20mm tooling (Autodesk Fusion 360 design; units mm, degrees)
Autodesk Fusion 360 part; units mm, degrees
note: some values were not read from the file. Chosen so that the rebuilt part matches the saved one: which pieces of a blend or face edit are solid. Set by a fixed rule: which sketch regions a step uses.
sketch "Sketch1" plane through (0, 0, 0) normal (0, 1, 0) x (1, 0, 0)
  line L0 (0, 0) -> (144, 0)
  line L1 (144, -40) -> (0, -40)
  line L2 (0, -40) -> (0, 0)
  line L3 (0, -20) -> (144, -20)
  line L4 (0, 0) -> (10, 0)
  line L5 (144, 0) -> (140, 0)
  line L6 (10, 0) -> (36, 0)
  line L7 (36, -40) -> (62, -40)
  line L8 (62, 0) -> (88, 0)
  line L9 (88, -40) -> (114, -40)
  line L10 (114, 0) -> (140, 0)
  circle A0 centre (20, -20) radius 10
  circle A1 centre (46, -20) radius 10
  circle A2 centre (72, -20) radius 10
  circle A3 centre (124, -20) radius 10
  line L11 (134, -20) -> (144, -20)
  line L12 (144, -40) -> (144, 0)
  circle A4 centre (98, -20) radius 10
  line L13 (0, 0) -> (144, 0)
  line L14 (144, 0) -> (144, -5)
  line L15 (144, -5) -> (0, -5)
  line L16 (0, -5) -> (0, 0)
  line L17 (0, -40) -> (5, -40)
  line L18 (5, -40) -> (5, 0)
  line L19 (5, 0) -> (0, 0)
  line L20 (0, 0) -> (0, -40)
  line L21 (144, -40) -> (139, -40)
  line L22 (139, -40) -> (139, 0)
  line L23 (139, 0) -> (144, 0)
  line L24 (144, 0) -> (144, -40)
  dimension "d8" = 20
  dimension "d9" = 20
  dimension "d10" = 20
  dimension "d12" = 20
  dimension "d15" = 20
  dimension "d16" = 5
  dimension "d17" = 5
  constraint horizontal L0
  constraint horizontal L1
  constraint vertical L2
  constraint coincident L0.start L2.end
  constraint midpoint L2 L3.start
  constraint coincident L0 L4.end
  constraint perpendicular L2 L4
  constraint coincident L0 L5.end
  constraint coincident L1 L7.start
  constraint coincident L0 L8.start
  constraint coincident L1 L9.start
  constraint coincident L0 L10.start
  constraint coincident A3 L11.start
  constraint coincident L3 L11.start
  constraint coincident L1 L12.start
  constraint vertical L12
  constraint horizontal L13
  constraint vertical L14
  constraint horizontal L15
  constraint vertical L16
  constraint horizontal L17
  constraint vertical L18
  constraint horizontal L19
  constraint vertical L20
  constraint midpoint L4 L18.end
  constraint horizontal L21
  constraint vertical L22
  constraint horizontal L23
  constraint vertical L24
  measures "d8" diameter of A0
  measures "d9" diameter of A1
  measures "d10" diameter of A2
  measures "d12" diameter of A3
  measures "d15" diameter of A4
  measures "d16" distance of L0.start L15.end
  measures "d17" distance of L1.start L21.end
extrude "Extrude1" add sketch "Sketch1" along normal blind 5 contours L0 L2 L4 L13 L15 L16 L18 L19 L20 | L0 L4 L6 L8 L10 L13 L15 L18 L22 | L2 L3 L15 L18 L20 | L3 A0 A1 A2 A3 L11 A4 L15 L18 L22 | L1 L2 L3 L17 L18 L20 | L0 L5 L10 L12 L13 L14 L15 L22 L23 L24 | L3 L11 L12 L15 L22 L24 | L1 L3 L7 L9 A0 A1 A2 A3 L11 A4 L18 L22 | L1 L3 L11 L12 L21 L22 L24
fillet "Fillet1" radius 2 10 edges at (10.6767, 5, 16.3838) (36.6767, 5, 16.3838) (62.6767, 5, 16.3838) (88.6767, 5, 16.3838) (114.6767, 5, 16.3838) (10.6767, 0, 16.3838) (36.6767, 0, 16.3838) (62.6767, 0, 16.3838) (88.6767, 0, 16.3838) (114.6767, 0, 16.3838)
fillet "Fillet2" radius 2 2 edges at (72, 5, 40) (72, 0, 40)
sketch "Sketch2" plane through (0, 0, 0) normal (0, -1, 0) x (1, 0, 0)
  circle A0 centre (124, 20) radius 12
  circle A1 centre (72, 20) radius 12
  circle A2 centre (20, 20) radius 12
  line L0 (144, 38) -> (0, 38)
  line L1 (0, 38) -> (0, 0)
  line L2 (0, 0) -> (144, 0)
  line L3 (144, 0) -> (144, 38)
  circle A3 centre (46, 20) radius 12
  circle A4 centre (98, 20) radius 12
  line L4 (0, 0) -> (144, 0)
  line L5 (144, 0) -> (144, 5)
  line L6 (144, 5) -> (0, 5)
  line L7 (0, 5) -> (0, 0)
  line L8 (0, 0) -> (5, 0)
  line L9 (5, 0) -> (5, 38)
  line L10 (5, 38) -> (0, 38)
  line L11 (0, 38) -> (0, 0)
  line L12 (144, 0) -> (139, 0)
  line L13 (139, 0) -> (139, 38)
  line L14 (139, 38) -> (144, 38)
  line L15 (144, 38) -> (144, 0)
  dimension "d22" = 5
  dimension "d23" = 5
  dimension "d24" = 5
  constraint horizontal L4
  constraint vertical L5
  constraint horizontal L6
  constraint vertical L7
  constraint coincident L1.end L2.start
  constraint horizontal L8
  constraint vertical L9
  constraint horizontal L10
  constraint vertical L11
  constraint horizontal L12
  constraint vertical L13
  constraint horizontal L14
  constraint vertical L15
  measures "d22" distance of L1.end L6.end
  measures "d23" distance of L1.end L8.end
  measures "d24" distance of L2.end L12.end
extrude "Extrude2" add sketch "Sketch2" along normal blind 5 contours L0 L3 L6 L13 L14 L15 | L2 L3 L4 L5 L6 L12 L13 L15 | L0 L1 L6 L9 L10 L11 | L2 L4 L6 L9 L13 | L1 L2 L4 L6 L7 L8 L9 L11
fillet "Fillet3" radius 100 2 edges at (2.5, -5, 38) (141.5, -5, 38)
sketch "Sketch3" plane through (0, -5, 0) normal (0, -1, 0) x (1, 0, 0)
  line L0 (144, 6.775) -> (139, 6.775)
  line L1 (139, 6.775) -> (139, 5)
  line L2 (139, 5) -> (5, 5)
  line L3 (5, 5) -> (5, 6.775)
  line L4 (5, 6.775) -> (0, 6.775)
  line L5 (0, 6.775) -> (0, 0)
  line L6 (0, 0) -> (144, 0)
  line L7 (144, 0) -> (144, 6.775)
  line L8 (72, 0) -> (72, 5)
  line L9 (72, 5) -> (82, 5)
  line L10 (82, 5) -> (82, 0)
  line L11 (82, 0) -> (72, 0)
  line L12 (72, 0) -> (72, 5)
  line L13 (72, 0) -> (62, 0)
  line L14 (62, 0) -> (62, 5)
  line L15 (62, 5) -> (72, 5)
  line L16 (72, 5) -> (72, 0)
  line L17 (5, 5) -> (25, 5)
  line L18 (25, 5) -> (25, 0)
  line L19 (25, 0) -> (5, 0)
  line L20 (5, 0) -> (5, 5)
  line L21 (139, 5) -> (119, 5)
  line L22 (119, 5) -> (119, 0)
  line L23 (119, 0) -> (139, 0)
  line L24 (139, 0) -> (139, 5)
  dimension "d28" = 10
  dimension "d29" = 10
  dimension "d30" = 20
  dimension "d31" = 20
  constraint midpoint L6 L8.start
  constraint midpoint L2 L8.end
  constraint horizontal L9
  constraint vertical L10
  constraint horizontal L11
  constraint vertical L12
  constraint horizontal L13
  constraint vertical L14
  constraint horizontal L15
  constraint vertical L16
  constraint horizontal L17
  constraint vertical L18
  constraint horizontal L19
  constraint vertical L20
  constraint coincident L2.end L3.start
  constraint horizontal L21
  constraint vertical L22
  constraint horizontal L23
  constraint vertical L24
  constraint coincident L1.end L2.start
  measures "d28" distance of L8.end L9.end
  measures "d29" distance of L8.start L13.end
  measures "d30" distance of L2.end L17.end
  measures "d31" distance of L1.end L21.end
extrude "Extrude3" add sketch "Sketch3" along normal blind 10 contours L2 L6 L21 L22 L23 L24 | L2 L6 L8 L9 L10 L11 L12 L16 | L2 L6 L8 L12 L13 L14 L15 L16 | L2 L6 L17 L18 L19 L20
fillet "Fillet4" radius 10 6 edges at (5, -15, 2.5) (25, -15, 2.5) (62, -15, 2.5) (82, -15, 2.5) (119, -15, 2.5) (139, -15, 2.5)
sketch "Sketch4" plane through (0, 0, 5) normal (0, 0, 1) x (1, 0, 0)
  arc A0 (119, -5) -> (139, -5) centre (129, -5) ccw
  line L0 (139, -5) -> (139, 0)
  line L1 (139, 0) -> (5, 0)
  line L2 (5, 0) -> (5, -5)
  arc A1 (5, -5) -> (25, -5) centre (15, -5) ccw
  line L3 (25, -5) -> (62, -5)
  arc A2 (62, -5) -> (82, -5) centre (72, -5) ccw
  line L4 (82, -5) -> (119, -5)
  line L5 (15, -15) -> (15, 0)
  line L6 (72, -15) -> (72, 0)
  line L7 (129, -15) -> (129, 0)
  line L8 (5, -5) -> (139, -5)
  circle A3 centre (15, -5) radius 1.5
  circle A4 centre (10, -5) radius 1.5
  circle A5 centre (20, -5) radius 1.5
  circle A6 centre (72, -5) radius 1.5
  line L9 (62, -5) -> (82, -5)
  line L10 (62, -5) -> (67, -5)
  line L11 (82, -5) -> (77, -5)
  circle A7 centre (67, -5) radius 1.5
  circle A8 centre (77, -5) radius 1.5
  line L12 (119, -5) -> (139, -5)
  circle A9 centre (129, -5) radius 1.5
  line L13 (119, -5) -> (129, -5)
  circle A10 centre (124, -5) radius 1.5
  line L14 (139, -5) -> (129, -5)
  circle A11 centre (134, -5) radius 1.5
  line L15 (72, -5) -> (72, -15)
  circle A12 centre (72, -10) radius 1.5
  line L16 (15, -15) -> (15, -5)
  circle A13 centre (15, -10) radius 1.5
  line L17 (129, -15) -> (129, -5)
  circle A14 centre (129, -10) radius 1.5
  circle A15 centre (15, 0) radius 1.5
  circle A16 centre (72, 0) radius 1.5
  circle A17 centre (129, 0) radius 1.5
  dimension "d35" = 3
  dimension "d36" = 3
  dimension "d37" = 3
  dimension "d38" = 3
  dimension "d39" = 5
  dimension "d40" = 3
  dimension "d41" = 3
  dimension "d42" = 3
  dimension "d43" = 3
  dimension "d44" = 3
  dimension "d45" = 3
  dimension "d46" = 3
  dimension "d47" = 3
  dimension "d48" = 3
  dimension "d49" = 3
  dimension "d50" = 3
  constraint midpoint A1 L5.start
  constraint coincident L1 L5.end
  constraint midpoint A2 L6.start
  constraint midpoint L1 L6.end
  constraint midpoint A0 L7.start
  constraint coincident L1 L7.end
  constraint vertical L7
  constraint coincident L2.end A1.start
  constraint coincident A0.end L0.start
  constraint concentric A1 A3
  constraint coincident L8 A4.centre
  constraint concentric A2 A6
  constraint coincident L3.end A2.start
  constraint coincident A2.end L4.start
  constraint coincident L9 L10.end
  constraint perpendicular L6 L10
  constraint coincident L10.end A7.centre
  constraint coincident L11.end A8.centre
  constraint coincident A0.start L4.end
  constraint concentric A0 A9
  constraint coincident A0.centre A9.centre
  constraint midpoint L13 A10.centre
  constraint midpoint L14 A11.centre
  constraint coincident A2.centre A6.centre
  constraint midpoint L15 A12.centre
  constraint coincident A1.centre A3.centre
  constraint midpoint L16 A13.centre
  constraint midpoint L17 A14.centre
  constraint coincident L5.end A15.centre
  constraint coincident L6.end A16.centre
  constraint coincident L7.end A17.centre
  measures "d35" diameter of A3
  measures "d36" diameter of A4
  measures "d37" diameter of A5
  measures "d38" diameter of A6
  measures "d39" distance of A2.end L11.end
  measures "d40" diameter of A7
  measures "d41" diameter of A8
  measures "d42" diameter of A9
  measures "d43" diameter of A10
  measures "d44" diameter of A11
  measures "d45" diameter of A12
  measures "d46" diameter of A13
  measures "d47" diameter of A14
  measures "d48" diameter of A15
  measures "d49" diameter of A16
  measures "d50" diameter of A17
extrude "Extrude4" cut sketch "Sketch4" along normal blind 20 contours L8 L12 L13 A10 | L8 L12 L13 A10 | L7 L17 A14 | L7 L17 A14 | L8 L9 L11 A8 | L8 L9 L11 A8 | L8 L12 L14 A11 | L8 L12 L14 A11 | L6 L15 A12 | L6 L15 A12 | L7 L8 L12 A9 L13 | L7 L8 L12 A9 L13 L17 | L1 L7 A17 | L1 A17 | L7 L8 L12 A9 L14 L17 | L8 L9 L10 A7 | L8 L9 L10 A7 | L6 L8 A6 L9 L15 | L6 L8 A6 L9 | L7 L8 L12 A9 L14 | L1 L7 A17 | L8 A5 | L8 A5 | L6 L8 A6 L9 L15 | L6 L8 A6 L9 | L1 L6 A16 | L1 A16 | L5 L16 A13 | L5 L16 A13 | L1 L6 A16 | L8 A4 | L8 A4 | L5 L8 A3 L16 | L5 L8 A3 | L1 L5 A15 | L1 A15 | L1 L5 A15 | L5 L8 A3 L16 | L5 L8 A3
extrude "Extrude5" cut sketch "Sketch4" against normal blind 10 contours L8 L12 L13 A10 | L8 L12 L13 A10 | L7 L17 A14 | L7 L17 A14 | L8 L9 L11 A8 | L8 L9 L11 A8 | L8 L12 L14 A11 | L8 L12 L14 A11 | L6 L15 A12 | L6 L15 A12 | L7 L8 L12 A9 L13 | L7 L8 L12 A9 L13 L17 | L1 L7 A17 | L1 A17 | L7 L8 L12 A9 L14 L17 | L8 L9 L10 A7 | L8 L9 L10 A7 | L6 L8 A6 L9 L15 | L6 L8 A6 L9 | L7 L8 L12 A9 L14 | L1 L7 A17 | L8 A5 | L8 A5 | L6 L8 A6 L9 L15 | L6 L8 A6 L9 | L1 L6 A16 | L1 A16 | L5 L16 A13 | L5 L16 A13 | L1 L6 A16 | L8 A4 | L8 A4 | L5 L8 A3 L16 | L5 L8 A3 | L1 L5 A15 | L1 A15 | L1 L5 A15 | L5 L8 A3 L16 | L5 L8 A3
sketch "Sketch5" plane through (0, 0, 0) normal (0, 0, -1) x (-1, 0, 0)
  arc A0 (-139, -5) -> (-119, -5) centre (-129, -5) ccw
  line L0 (-119, -5) -> (-82, -5)
  arc A1 (-82, -5) -> (-62, -5) centre (-72, -5) ccw
  line L1 (-62, -5) -> (-25, -5)
  arc A2 (-25, -5) -> (-5, -5) centre (-15, -5) ccw
  line L2 (-5, -5) -> (0, -5)
  line L3 (0, -5) -> (0, 5)
  line L4 (0, 5) -> (-144, 5)
  line L5 (-144, 5) -> (-144, -5)
  line L6 (-144, -5) -> (-139, -5)
  circle A3 centre (-15, -10) radius 1.5
  circle A4 centre (-72, -5) radius 1.5
  circle A5 centre (-129, -5) radius 1.5
  circle A6 centre (-15, 0) radius 1.5
  circle A7 centre (-124, -5) radius 1.5
  circle A8 centre (-67, -5) radius 1.5
  circle A9 centre (-10, -5) radius 1.5
  circle A10 centre (-15, -5) radius 1.5
  circle A11 centre (-72, -10) radius 1.5
  circle A12 centre (-129, -10) radius 1.5
  circle A13 centre (-72, 0) radius 1.5
  circle A14 centre (-129, 0) radius 1.5
  circle A15 centre (-134, -5) radius 1.5
  circle A16 centre (-77, -5) radius 1.5
  circle A17 centre (-20, -5) radius 1.5
sketch "Sketch6" plane through (0, 0, 5) normal (0, 0, 1) x (1, 0, 0)
  circle A0 centre (72, 0) radius 3
  circle A1 centre (67, -5) radius 3
  circle A2 centre (77, -5) radius 3
  circle A3 centre (72, -10) radius 3
  circle A4 centre (15, 0) radius 3
  circle A5 centre (10, -5) radius 3
  circle A6 centre (20, -5) radius 3
  circle A7 centre (15, -10) radius 3
  circle A8 centre (129, 0) radius 3
  circle A9 centre (124, -5) radius 3
  circle A10 centre (134, -5) radius 3
  circle A11 centre (129, -10) radius 3
  point P0 (72, 0)
  point P1 (67, -5)
  point P2 (77, -5)
  point P3 (72, -10)
  point P4 (15, 0)
  point P5 (10, -5)
  point P6 (15, -10)
  point P7 (129, 0)
  point P8 (124, -5)
  point P9 (134, -5)
  point P10 (129, -10)
  dimension "d55" = 6
  dimension "d56" = 6
  dimension "d57" = 6
  dimension "d58" = 6
  dimension "d59" = 6
  dimension "d60" = 6
  dimension "d61" = 6
  dimension "d62" = 6
  dimension "d63" = 6
  dimension "d64" = 6
  dimension "d65" = 6
  dimension "d66" = 6
  constraint coincident P0 A0.centre
  constraint coincident P1 A1.centre
  constraint coincident P2 A2.centre
  constraint coincident P3 A3.centre
  constraint coincident P4 A4.centre
  constraint coincident P5 A5.centre
  constraint coincident P6 A7.centre
  constraint coincident P7 A8.centre
  constraint coincident P8 A9.centre
  constraint coincident P9 A10.centre
  constraint coincident P10 A11.centre
  measures "d55" diameter of A0
  measures "d56" diameter of A1
  measures "d57" diameter of A2
  measures "d58" diameter of A3
  measures "d59" diameter of A4
  measures "d60" diameter of A5
  measures "d61" diameter of A6
  measures "d62" diameter of A7
  measures "d63" diameter of A8
  measures "d64" diameter of A9
  measures "d65" diameter of A10
  measures "d66" diameter of A11
chamfer "Chamfer1" distance 3 angle 45 3 edges at (13.6015, -4.4576, 5) (70.6015, -4.4576, 5) (127.6015, -4.4576, 5)
extrude "Extrude6" cut sketch "Sketch6" along normal blind 20
extrude "Extrude7" cut sketch "Sketch6" against normal blind 3.5
fillet "Fillet5" radius 2 3 edges at (15, -15, 5) (72, -15, 5) (129, -15, 5)
